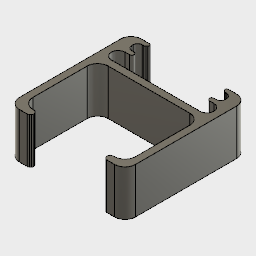
clip h-bridge (Autodesk Fusion 360 design; units mm, degrees)
Autodesk Fusion 360 part; units mm, degrees
note: some values were not read from the file. Set by a fixed rule: which sketch regions a step uses.
sketch "Sketch1" plane through (0, 0, 0) normal (0, 1, 0) x (1, 0, 0)
  line L0 (-8.25, 14.8) -> (-12.75, 14.8)
  line L1 (-12.75, 14.8) -> (-8.25, 14.8)
  line L2 (-8.25, 13.8) -> (-10.25, 13.8)
  line L3 (-11.25, -10.5) -> (-8, -10.5)
  line L4 (-8, -10.5) -> (-8, -12)
  line L5 (-8, -12) -> (-12.75, -12)
  line L6 (-8.25, 13.8) -> (-8.25, 14.8)
  line L7 (-10.25, 13.8) -> (-10.25, 11.5)
  line L8 (-10.25, 11.5) -> (-8.25, 11.5)
  line L9 (-8.25, 11.5) -> (-8.25, 10.5)
  line L10 (-8.25, 10.5) -> (-11.25, 10.5)
  line L11 (-12.75, 14.8) -> (-12.75, -12)
  line L12 (0, 7.5) -> (-11.25, 7.5)
  line L13 (-11.25, 7.5) -> (-11.25, 10.5)
  line L14 (0, 7.5) -> (0, 6)
  line L15 (0, 6) -> (-11.25, 6)
  line L16 (-11.25, 6) -> (-11.25, -10.5)
  dimension "d1" = 2.3
  dimension "d2" = 1
  dimension "d3" = 1
  dimension "d5" = 2
  dimension "d8" = 1.5
  dimension "d11" = 8
  dimension "d13" = 10.5
  dimension "d14" = 10.5
  dimension "d17" = 1
  dimension "d28" = 1.5
  dimension "d29" = 1.5
  dimension "d30" = 3
  dimension "d34" = 10.25
  measures "d1" distance of L2.end L7.end
  measures "d2" distance of L8.end L9.end
  measures "d3" distance of L0.start L2.start
  measures "d5" distance of L2.start L2.end
  measures "d8" distance of L3.end L4.end
  measures "d11" distance of origin L4.end
  measures "d13" distance of origin L9.end
  measures "d14" distance of origin L3.end
  measures "d17" distance of L7.end L10.end
  measures "d28" distance of L3.start L5.end
  measures "d29" distance of L12.start L14.end
  measures "d30" distance of L10 L12
  measures "d34" distance of origin L2.end
extrude "Extrude1" add sketch "Sketch1" along normal blind 10 makes body 1
chamfer "Chamfer1" distance 0.5 angle 45 3 edges at (-8.25, 5, -13.8) (-8, 5, 12) (-8, 5, 10.5) on bodies 1
fillet "Fillet1" radius 0.5 6 edges at (-8, 5, 11.5) (-8, 5, 11) (-8.5, 5, 12) (-8.5, 5, 10.5) (-8.25, 5, -14.3) (-8.75, 5, -13.8) on bodies 1
fillet "Fillet2" radius 2.3 4 edges at (-12.75, 5, 12) (-12.75, 5, -14.8) (-11.25, 5, -6) (-11.25, 5, 10.5) on bodies 1
fillet "Fillet3" radius 0.5 3 edges at (-8.25, 5, -14.8) (-8.25, 5, -11.5) (-8.25, 5, -10.5) on bodies 1
fillet "Fillet4" radius 1 2 edges at (-10.25, 5, -13.8) (-10.25, 5, -11.5) on bodies 1
fillet "Fillet5" radius 1.5 2 edges at (-11.25, 5, -10.5) (-11.25, 5, -7.5) on bodies 1
mirror "Mirror1" about plane through (0, 0, -7.5) normal (1, 0, 0) of bodies 1 makes body 2
combine "Combine1" operation add target body 1 tool bodies 2
